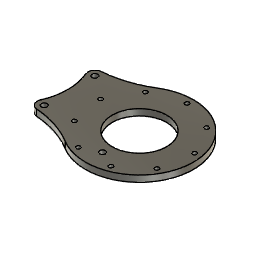
电机支架面板1.1 v2 (Autodesk Fusion 360 design; units mm, degrees)
Autodesk Fusion 360 part; units mm, degrees
sketch "草图1" plane through (0, 0, 0) normal (0, 0, 1) x (1, 0, 0)
  circle A0 centre (0, 0) radius 21.5
  circle A1 centre (0, 0) radius 37.5 construction
  circle A2 centre (0, 0) radius 42.5
  line L0 (0, 0) -> (0, 56.853) construction
  circle A3 centre (0, 37.5) radius 1.65
  circle A4 centre (-24.1045, 28.7267) radius 1.65
  circle A5 centre (-36.9303, 6.5118) radius 1.65
  circle A6 centre (-32.476, -18.75) radius 1.65
  circle A7 centre (-12.8258, -35.2385) radius 1.65
  circle A8 centre (12.8258, -35.2385) radius 1.65
  circle A9 centre (32.476, -18.75) radius 1.65
  circle A10 centre (36.9303, 6.5118) radius 1.65
  circle A11 centre (24.1045, 28.7267) radius 1.65
  line L1 (0, 0) -> (0, -49) construction
  circle A12 centre (0, -29) radius 2.2361
  dimension "d1" = 43
  dimension "d2" = 75
  dimension "d3" = 85
  dimension "d4" = 3.3
  dimension "d6" = 360
  dimension "d8" = 29
  constraint coincident A0.centre A1.centre
  constraint concentric A0 A1
  constraint concentric A0 A2
  constraint vertical L0
  constraint coincident A1 A3.centre
  constraint coincident L0 A3.centre
  constraint parallel L0 L1
  constraint coincident L1 A12.centre
  measures "d1" diameter of A0
  measures "d2" diameter of A1
  measures "d3" diameter of A2
  measures "d4" diameter of A3
  measures "d8" distance of A0.centre A12.centre
extrude "拉伸1" add sketch "草图1" along normal blind 5
sketch "草图5" plane through (0, 0, 0) normal (0, 0, 1) x (1, 0, 0)
  circle A0 centre (-55, 20) radius 2.25
  circle A1 centre (-55, -20) radius 2.25
  circle A2 centre (-55, 20) radius 5.5
  circle A3 centre (-55, -20) radius 5.5
  circle A4 centre (0, 0) radius 42.5
  circle A5 centre (-61.2801, 100.2547) radius 75
  circle A6 centre (-61.2801, -100.2547) radius 75
  circle A7 centre (-101.3708, 0) radius 45
  dimension "d19" = 40
  dimension "d20" = 4.5
  dimension "d21" = 4.5
  dimension "d22" = 20
  dimension "d23" = 11
  dimension "d24" = 11
  dimension "d25" = 85
  dimension "d26" = 150
  dimension "d27" = 55
  dimension "d28" = 150
  dimension "d29" = 90
  constraint vertical A0.centre A1.centre
  constraint concentric A0 A2
  constraint concentric A1 A3
  constraint coincident A4.centre origin
  constraint tangent A2 A5
  constraint tangent A4 A5
  constraint tangent A3 A6
  constraint tangent A4 A6
  constraint tangent A2 A7
  constraint tangent A3 A7
  measures "d19" vertical distance of A0.centre A1.centre
  measures "d20" diameter of A0
  measures "d21" diameter of A1
  measures "d22" vertical distance of A4.centre A0.centre
  measures "d23" diameter of A2
  measures "d24" diameter of A3
  measures "d25" diameter of A4
  measures "d26" diameter of A5
  measures "d27" horizontal distance of A0.centre A4.centre
  measures "d28" diameter of A6
  measures "d29" diameter of A7
extrude "拉伸3" add sketch "草图5" along normal blind 5 contours A2 | A2 A3 A4 A5 A6 A7 | A3
